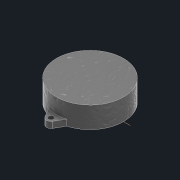
# Autodesk Inventor part: speaker
Saved by Autodesk Inventor 2022 (Build 260153000, 153)
## iProperties
Created: 2022-01-13
Part Number: speaker
Material: Generic
Document SubType Name: Modeling
Designer: Andres
Density: 1 g/cm^3
Appearance: Fine Textured - Black
Author: Andres
Autodesk Inventor part; units mm, degrees
ref_plane "YZ Plane" through (0, 0, 0) normal (1, 0, 0) x (0, 1, 0)
ref_plane "XZ Plane" through (0, 0, 0) normal (0, 1, 0) x (-1, 0, 0)
ref_plane "XY Plane" through (0, 0, 0) normal (0, 0, 1) x (1, 0, 0)
sketch "Sketch1" plane through (0, 0, 0) normal (0, 1, 0) x (-1, 0, 0)
  circle A0 centre (0, 0) radius 22
  circle A1 centre (0, -25.5) radius 3
  line L0 (2.5981, -27) -> (5.9598, -21.1774)
  line L1 (-2.5981, -27) -> (-5.9598, -21.1774)
  line L2 (30.8, 0) -> (-30.8, 0) projected
  circle A2 centre (0, 25.5) radius 3
  line L3 (2.5981, 27) -> (5.9598, 21.1774)
  line L4 (-2.5981, 27) -> (-5.9598, 21.1774)
  point P0 (5.9598, 21.1774)
  point P1 (-5.9598, 21.1774)
  dimension "d0" = 44
  dimension "d1" = 60
  dimension "d2" = 6
  dimension "d3" = 51
  constraints: 8 end point, 6 point on circle, 5 symmetric about line, 3 centre point, 3 coincident, 2 tangent, 1 equal length, 1 vertical alignment, 1 other
  measures "d0" diameter of A0
  measures "d1" angle of L0 L1
  measures "d2" diameter of A1
  measures "d3" distance of A2.centre A1.centre
extrude "Extrusion1" add sketch "Sketch1" along normal blind 14 contours L2 A0 | A0 L2
extrude "Extrusion2" add sketch "Sketch1" along normal blind 4 contours A0 L4 A2 L3 | L0 A1 L1 A0 | A2 | A1
hole "Hole1" at (0, 0, -25.5) at (0, 0, 25.5) direction (0, 1, 0) diameter 3.4 depth 4 clearance for "Socket Head Cap Screw ISO 4762" size "M3" standard "ISO"
sketch "Sketch2" plane through (0, 0, 0) normal (0, 1, 0) x (1, 0, 0)
  circle A0 centre (0, 0) radius 4
  dimension "d15" = 8
  constraints: 1 centre point, 1 coincident
  measures "d15" diameter of A0
extrude "Extrusion3" cut sketch "Sketch2" along normal blind 3
body "Solid1"
